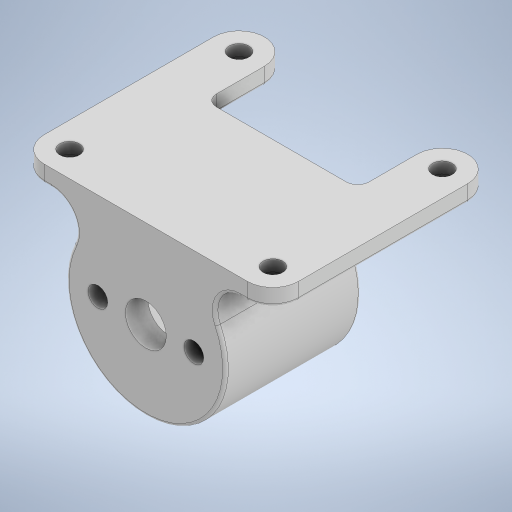
# Autodesk Inventor part: v4motormount
Saved by Autodesk Inventor 2024.2 (Build 282272000, 272)
## iProperties
Created: 2024-02-10
Part Number: v4motormount
Material: Generic
Document SubType Name: Modeling
Designer: Eric
Density: 1 g/cm^3
Appearance: Default
Author: Eric
Autodesk Inventor part; units mm, degrees
ref_plane "YZ Plane" through (0, 0, 0) normal (1, 0, 0) x (0, 1, 0)
ref_plane "XY Plane" through (0, 0, 0) normal (0, 0, 1) x (1, 0, 0)
sketch "Sketch1" plane through (0, 0, 0) normal (0, 0, 1) x (1, 0, 0)
  circle A0 centre (-8.5, 0) radius 1.75
  circle A1 centre (8.5, 0) radius 1.75
  circle A2 centre (0, 0) radius 3.625
  circle A3 centre (0, 0) radius 14.1
  line L0 (0, 20.8064) -> (0, -22.8434) construction
  dimension "d0" = 7.25
  dimension "d1" = 3.5
  dimension "d2" = 17
  dimension "d3" = 28.2
  constraints: 4 centre point, 2 coincident, 2 end point, 2 horizontal alignment, 1 equal radius, 1 point on line, 1 vertical, 1 other
  measures "d0" diameter of A2
  measures "d1" diameter of A0
  measures "d2" distance of A0.centre A1.centre
  measures "d3" diameter of A3
extrude "Extrusion1" add sketch "Sketch1" against normal blind 4
sketch "Sketch2" plane through (0, 0, -4) normal (0, 0, -1) x (-1, 0, 0)
  circle A0 centre (0, 0) radius 14.1 projected
  circle A1 centre (0, 0) radius 12.6
  dimension "d6" = 25.2
  constraints: 1 centre point, 1 coincident
  measures "d6" diameter of A1
extrude "Extrusion2" add sketch "Sketch2" along normal blind 20
ref_plane "Work Plane1" through (0, 12.6, 0) normal (0, 1, 0) x (-1, 0, 0)
sketch "Sketch3" plane through (0, 12.6, 0) normal (0, 1, 0) x (-1, 0, 0)
  line L0 (-22.5, -24) -> (22.5, -24) construction
  line L1 (22.5, -24) -> (22.5, 0) construction
  line L2 (22.5, 0) -> (-22.5, 0) construction
  line L3 (-22.5, 0) -> (-22.5, -24) construction
  line L4 (-14.1, -24) -> (14.1, -24) projected
  line L5 (14.1, 0) -> (-14.1, 0) projected
  circle A0 centre (18, -4.5) radius 1.75
  circle A1 centre (-18, -4.5) radius 1.75
  circle A2 centre (-18, -34.5) radius 1.75
  circle A3 centre (18, -34.5) radius 1.75
  circle A4 centre (18, -4.5) radius 4.5
  circle A5 centre (18, -34.5) radius 4.5
  circle A6 centre (-18, -4.5) radius 4.5
  circle A7 centre (-18, -34.5) radius 4.5
  line L6 (22.5, -34.5) -> (22.5, -4.5)
  line L7 (18, 0) -> (-18, 0)
  line L8 (-22.5, -34.5) -> (-22.5, -4.5)
  line L9 (13.5, -34.5) -> (13.5, -24)
  line L10 (-13.5, -24) -> (-13.5, -34.5)
  line L11 (13.5, -24) -> (-13.5, -24)
  point P0 (0, 0)
  point P1 (0, 0)
  dimension "d14" = 45
  dimension "d15" = 22.5
  dimension "d16" = 3.5
  dimension "d17" = 4.5
  dimension "d18" = 4.5
  dimension "d19" = 4.5
  dimension "d31" = 30
  constraints: 20 end point, 8 centre point, 8 point on circle, 8 tangent, 5 perpendicular, 4 coincident, 4 point on line, 3 collinear, 3 equal radius, 2 horizontal alignment, 2 vertical alignment, 1 horizontal, 1 midpoint, 1 parallel, 1 vertical
  measures "d14" distance between parallel lines of L3 L1
  measures "d15" distance from line of point (0, 0) L3
  measures "d16" diameter of A0
  measures "d17" distance from line of L2 A0.centre
  measures "d18" distance from line of L1 A0.centre
  measures "d19" distance from line of L3 A2.centre
  measures "d31" distance of A0.centre A3.centre
extrude "Extrusion6" add sketch "Sketch3" along normal blind 3
sketch "Sketch6" plane through (0, 12.6, 0) normal (0, -1, 0) x (1, 0, 0)
  circle A0 centre (18, -4.5) radius 1.75 projected
  circle A1 centre (18, -4.5) radius 2.625
  circle A2 centre (18, -34.5) radius 1.75 projected
  circle A3 centre (18, -34.5) radius 2.625
  circle A4 centre (-18, -4.5) radius 1.75 projected
  circle A5 centre (-18, -4.5) radius 2.625
  circle A6 centre (-18, -34.5) radius 1.75 projected
  circle A7 centre (-18, -34.5) radius 2.625
  point P0 (0, 0)
  dimension "d46" = 5.25
  constraints: 4 centre point, 4 coincident, 3 equal radius
  measures "d46" diameter of A1
extrude "Extrusion7" cut sketch "Sketch6" against normal blind 1 contours A0 | A1 | A2 | A3 | A4 | A5 | A6 | A7
fillet "Fillet3" radius 4.5 4 edges at (6.3285, 12.6, -2) (6.3285, 12.6, -14) (-6.3285, 12.6, -2) (-6.3285, 12.6, -14)
sketch "Sketch7" plane through (0, 0, 0) normal (0, 1, 0) x (-1, 0, 0)
  line L0 (-14.1, -24) -> (14.1, -24) projected
  line L1 (22.5, -34.5) -> (22.5, -4.5) projected
  line L2 (22.5, -24) -> (-22.5, -24)
  line L3 (-22.5, -4.5) -> (-22.5, -34.5) projected
  line L4 (22.5, -24) -> (22.5, -39)
  line L5 (22.5, -39) -> (-22.5, -39)
  line L6 (-22.5, -39) -> (-22.5, -24)
  arc A0 (-22.5, -34.5) -> (-16.7437, -38.8211) centre (-18, -34.5) ccw projected
  point P0 (0, 0)
  point P1 (-12.6928, -24)
  point P2 (12.6928, -24)
  constraints: 8 end point, 2 perpendicular, 2 point on line, 1 collinear, 1 horizontal, 1 tangent, 1 vertical
extrude "Extrusion8" cut sketch "Sketch7" along normal up to surface (12.6 mm away)
fillet "Fillet4" radius 2 4 edges at (13.5, 14.1, -24) (-13.5, 14.1, -24) (15.1218, 12.6, -24) (-15.1218, 12.6, -24)
fillet "Fillet5" radius 0.5 24 edges at (-21.182, 12.6, -1.318) (-17.3718, 12.6, 0) (-12.9313, 10.4908, 0) (13.7437, 3.1498, 0) (-3.1498, -13.7437, 0) (12.9313, 10.4908, 0) (17.3718, 12.6, 0) (21.182, 12.6, -1.318) (22.5, 12.6, -19.5) (18, 12.6, -39) (13.5, 12.6, -30.25) (12.9142, 12.0142, -24.5858) (-18, 12.6, -39) (-13.5, 12.6, -30.25) (-12.9142, 12.0142, -24.5858) (-22.5, 12.6, -19.5) (-12.2544, 8.4113, -24) (-15.0911, 12.2856, -24.9235) (-13.2422, 10.9266, -24.0269) (12.2544, 8.4113, -24) (13.2422, 10.9266, -24.0269) (15.0911, 12.2856, -24.9235) (-13.7437, 3.1498, -24) (3.1498, -13.7437, -24)
sketch "Sketch5" plane through (0, 0, 0) normal (0, 0, 1) x (1, 0, 0)
  circle A0 centre (-8.5, 0) radius 1.75 projected
  circle A1 centre (-8.5, 0) radius 2.625
  circle A2 centre (8.5, 0) radius 1.75 projected
  circle A3 centre (8.5, 0) radius 2.625
  point P0 (0, 0)
  dimension "d28" = 5.25
  constraints: 2 centre point, 2 coincident, 1 equal radius
  measures "d28" diameter of A1
body "Solid1"
